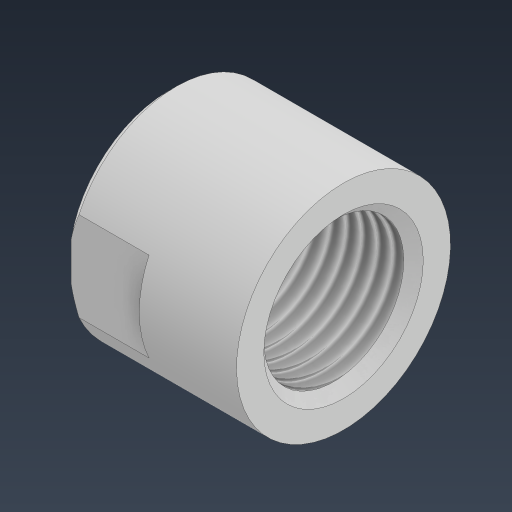
# Autodesk Inventor part: 3D Model
Saved by Autodesk Inventor 2024 (Build 280153000, 153)
## iProperties
Created: 2024-03-07
Part Number: 3D Model
Material: Genérico
Document SubType Name: Modeling
Designer: Administrator
Density: 1 g/cm^3
Appearance: Padrão
Author: Administrator
Autodesk Inventor part; units mm, degrees
ref_plane "YZ Plane" through (0, 0, 0) normal (1, 0, 0) x (0, 1, 0)
ref_plane "XZ Plane" through (0, 0, 0) normal (0, 1, 0) x (-1, 0, 0)
ref_plane "XY Plane" through (0, 0, 0) normal (0, 0, 1) x (1, 0, 0)
sketch "Esboço1" plane through (0, 0, 0) normal (0, 0, 1) x (1, 0, 0)
  line L0 (0, 0) -> (0, 27.5)
  line L1 (0, 27.5) -> (45, 27.5)
  line L2 (45, 27.5) -> (45, 18)
  line L3 (45, 18) -> (15, 18)
  line L4 (15, 18) -> (15, 20.5)
  line L5 (14, 21.5) -> (6, 21.5)
  line L6 (5, 20.5) -> (5, 0)
  line L7 (5, 0) -> (0, 0)
  arc A0 (6, 21.5) -> (5, 20.5) centre (6, 20.5) ccw
  arc A1 (15, 20.5) -> (14, 21.5) centre (14, 20.5) ccw
  point P0 (15, 21.5)
  point P1 (5, 21.5)
  point P2 (2.5, 0)
  dimension "d0" = 55
  dimension "d1" = 45
  dimension "d2" = 40
  dimension "d3" = 10
  dimension "d4" = 43
  dimension "d5" = 36
  dimension "d7" = 1
  constraints: 16 end point, 7 perpendicular, 4 point on circle, 4 point on line, 4 tangent, 2 centre point, 1 equal radius, 1 midpoint, 1 vertical
  measures "d0" diameter of L1 point (2.5, 0)
  measures "d1" distance between parallel lines of L0 L2
  measures "d2" distance between parallel lines of L2 L6
  measures "d3" distance between parallel lines of L6 L4
  measures "d4" diameter of L5 L7
  measures "d5" diameter of L3 L7
  measures "d7" radius of A0
revolve "Revolução1" add sketch "Esboço1" angle 360 about axis through (5, 0, 0) along (-1, 0, 0)
thread "Rosca1" size "M36x4" class "6H" standard "ANSI Metric M Profile" full length
chamfer "Chanfro1" distance 2.5 angle 45 1 edges at (45, -18, 0)
chamfer "Chanfro2" distance 2 angle 45 1 edges at (0, -27.5, 0)
sketch "Esboço2" plane through (0, 0, 0) normal (-1, 0, 0) x (0, 0, 1)
  line L0 (35, 15) -> (25, 15)
  line L1 (25, 15) -> (25, -15)
  line L2 (25, -15) -> (35, -15)
  line L3 (35, -15) -> (35, 15)
  line L4 (0, 0) -> (0, 48.3758) construction
  line L5 (-35, 15) -> (-25, 15)
  line L6 (-25, 15) -> (-25, -15)
  line L7 (-25, -15) -> (-35, -15)
  line L8 (-35, -15) -> (-35, 15)
  point P0 (25, 0)
  point P1 (35, 0)
  point P2 (30, -15)
  point P3 (-25, 0)
  point P4 (-35, 0)
  point P5 (-30, -15)
  dimension "d17" = 25
  dimension "d18" = 30
  dimension "d19" = 10
  constraints: 18 end point, 7 symmetric about line, 3 midpoint, 2 horizontal alignment, 2 parallel, 1 horizontal, 1 perpendicular, 1 vertical
  measures "d17" distance between parallel lines of L4 L1
  measures "d18" distance from line of point (30, -15) L0
  measures "d19" distance between parallel lines of L1 L3
extrude "Extrusão1" cut sketch "Esboço2" against normal blind 20
